Autodesk Inventor part; units mm, degrees
(part 2 of 2)
  arc A141 (-26.798, 74.2336) -> (-27.2062, 73.5932) centre (-26.3001, 73.4659) ccw
  arc A142 (-21.4794, 73.1947) -> (-22.0085, 74.2336) centre (-22.7699, 73.1916) ccw
  circle A143 centre (-25.9605, 73.338) radius 0.5161
  line L108 (-27.2062, 73.5932) -> (-27.2062, 72.1245)
  line L109 (-27.2062, 72.1245) -> (-24.3395, 72.1245)
  line L110 (-24.3395, 71.7056) -> (-28.3839, 71.7056)
  line L111 (-24.3395, 72.1245) -> (-24.3395, 71.7056)
  line L112 (-21.4733, 70.5884) -> (-21.4794, 73.1947)
  arc A144 (-23.3243, 25.8454) -> (-25.4322, 25.8454) centre (-24.3782, 17.6506) ccw
  arc A145 (-25.4322, 25.8454) -> (-26.7856, 25.3656) centre (-25.171, 22.9597) ccw
  arc A146 (-21.9961, 25.3656) -> (-23.3243, 25.8454) centre (-23.7019, 22.7218) ccw
  arc A147 (-21.4671, 24.3267) -> (-21.9961, 25.3656) centre (-22.7575, 24.3237) ccw
  arc A148 (-26.7856, 25.3656) -> (-27.1938, 24.7252) centre (-26.2877, 24.5979) ccw
  circle A149 centre (-25.9607, 24.5305) radius 0.545
  line L113 (-27.1938, 24.7252) -> (-27.1938, 23.2566)
  line L114 (-27.1938, 23.2566) -> (-24.3272, 23.2566)
  line L115 (-24.3272, 23.2566) -> (-24.3272, 22.8376)
  line L116 (-21.461, 21.7204) -> (-21.4671, 24.3267)
  line L117 (-26.0801, 20.1743) -> (-23.0926, 20.1813)
  arc A150 (-22.5618, 19.8544) -> (-21.3196, 20.5365) centre (-22.5875, 21.3734) ccw
  arc A151 (-23.0926, 20.1813) -> (-21.461, 21.7204) centre (-22.9431, 21.6573) ccw
  line L118 (-22.5618, 19.8544) -> (-25.5493, 19.8474)
  line L119 (-21.0597, 22.9429) -> (-21.0597, 21.4689)
  arc A152 (-21.3196, 20.5365) -> (-21.0597, 21.4689) centre (-22.9439, 21.4916) ccw
  line L120 (-19.9288, 22.9429) -> (-21.0597, 22.9429)
  arc A153 (-18.7198, 21.9341) -> (-19.9288, 22.9429) centre (-20.2582, 21.3193) ccw
  arc A154 (-18.5273, 18.7011) -> (-18.7198, 21.9341) centre (-23.4893, 20.0279) ccw
  arc A155 (-20.2704, 17.1911) -> (-18.5273, 18.7011) centre (-20.3549, 19.0497) ccw
  arc A156 (-25.5493, 19.8474) -> (-27.181, 18.3083) centre (-25.6988, 18.3715) ccw
  arc A157 (-26.0801, 20.1743) -> (-27.3224, 19.4922) centre (-26.0545, 18.6554) ccw
  line L121 (-24.3272, 22.8376) -> (-28.3715, 22.8376)
  arc A158 (-27.3224, 19.4922) -> (-27.5822, 18.5598) centre (-25.698, 18.5371) ccw
  line L122 (-27.5822, 17.0858) -> (-27.5822, 18.5598)
  arc A159 (-28.3715, 22.8376) -> (-30.1146, 21.3277) centre (-28.287, 20.979) ccw
  line L123 (-28.7131, 17.0858) -> (-27.5822, 17.0858)
  arc A160 (-30.1146, 21.3277) -> (-29.9221, 18.0946) centre (-25.1526, 20.0009) ccw
  arc A161 (-29.9221, 18.0946) -> (-28.7131, 17.0858) centre (-28.3837, 18.7095) ccw
  arc A162 (-25.3176, 14.1834) -> (-23.2097, 14.1834) centre (-24.2637, 22.3782) ccw
  arc A163 (-26.6458, 14.6631) -> (-25.3176, 14.1834) centre (-24.94, 17.307) ccw
  arc A164 (-23.2097, 14.1834) -> (-21.8563, 14.6631) centre (-23.4709, 17.0691) ccw
  arc A165 (-21.8563, 14.6631) -> (-21.4481, 15.3035) centre (-22.3542, 15.4308) ccw
  arc A166 (-27.1749, 15.702) -> (-26.6458, 14.6631) centre (-25.8844, 15.705) ccw
  circle A167 centre (-22.6938, 15.5587) radius 0.5161
  line L124 (-21.4481, 15.3035) -> (-21.4481, 16.7721)
  line L125 (-21.4481, 16.7721) -> (-24.3148, 16.7721)
  line L126 (-24.3148, 17.1911) -> (-20.2704, 17.1911)
  line L127 (-24.3148, 16.7721) -> (-24.3148, 17.1911)
  line L128 (-27.181, 18.3083) -> (-27.1749, 15.702)
  arc A168 (-46.4728, 48.6946) -> (-44.3649, 48.6946) centre (-45.4189, 56.8894) ccw
  arc A169 (-44.3649, 48.6946) -> (-43.0115, 49.1744) centre (-44.6261, 51.5803) ccw
  arc A170 (-47.801, 49.1744) -> (-46.4728, 48.6946) centre (-46.0952, 51.8182) ccw
  arc A171 (-48.33, 50.2133) -> (-47.801, 49.1744) centre (-47.0396, 50.2163) ccw
  arc A172 (-43.0115, 49.1744) -> (-42.6033, 49.8147) centre (-43.5094, 49.9421) ccw
  circle A173 centre (-43.8364, 50.0095) radius 0.545
  line L129 (-42.6033, 49.8147) -> (-42.6033, 51.2834)
  line L130 (-42.6033, 51.2834) -> (-45.4699, 51.2834)
  line L131 (-45.4699, 51.2834) -> (-45.4699, 51.7023)
  line L132 (-48.3361, 52.8196) -> (-48.33, 50.2133)
  line L133 (-43.717, 54.3657) -> (-46.7045, 54.3587)
  arc A174 (-47.2353, 54.6855) -> (-48.4775, 54.0034) centre (-47.2096, 53.1666) ccw
  arc A175 (-46.7045, 54.3587) -> (-48.3361, 52.8196) centre (-46.854, 52.8827) ccw
  line L134 (-47.2353, 54.6855) -> (-44.2478, 54.6925)
  line L135 (-48.7374, 51.5971) -> (-48.7374, 53.0711)
  arc A176 (-48.4775, 54.0034) -> (-48.7374, 53.0711) centre (-46.8532, 53.0484) ccw
  line L136 (-49.8683, 51.5971) -> (-48.7374, 51.5971)
  arc A177 (-51.0773, 52.6058) -> (-49.8683, 51.5971) centre (-49.5389, 53.2207) ccw
  arc A178 (-51.2698, 55.8389) -> (-51.0773, 52.6058) centre (-46.3078, 54.5121) ccw
  arc A179 (-49.5267, 57.3489) -> (-51.2698, 55.8389) centre (-49.4422, 55.4902) ccw
  arc A180 (-44.2478, 54.6925) -> (-42.6161, 56.2317) centre (-44.0983, 56.1685) ccw
  arc A181 (-43.717, 54.3657) -> (-42.4747, 55.0478) centre (-43.7426, 55.8846) ccw
  line L137 (-45.4699, 51.7023) -> (-41.4256, 51.7023)
  arc A182 (-42.4747, 55.0478) -> (-42.2149, 55.9801) centre (-44.0991, 56.0028) ccw
  line L138 (-42.2149, 57.4541) -> (-42.2149, 55.9801)
  arc A183 (-41.4256, 51.7023) -> (-39.6825, 53.2123) centre (-41.5101, 53.561) ccw
  line L139 (-41.084, 57.4541) -> (-42.2149, 57.4541)
  arc A184 (-39.6825, 53.2123) -> (-39.875, 56.4454) centre (-44.6445, 54.5391) ccw
  arc A185 (-39.875, 56.4454) -> (-41.084, 57.4541) centre (-41.4134, 55.8305) ccw
  arc A186 (-44.4795, 60.3566) -> (-46.5874, 60.3566) centre (-45.5334, 52.1618) ccw
  arc A187 (-43.1513, 59.8769) -> (-44.4795, 60.3566) centre (-44.8571, 57.233) ccw
  arc A188 (-46.5874, 60.3566) -> (-47.9408, 59.8769) centre (-46.3262, 57.4709) ccw
  arc A189 (-47.9408, 59.8769) -> (-48.349, 59.2365) centre (-47.4429, 59.1091) ccw
  arc A190 (-42.6222, 58.8379) -> (-43.1513, 59.8769) centre (-43.9127, 58.8349) ccw
  circle A191 centre (-47.1033, 58.9813) radius 0.5161
  line L140 (-48.349, 59.2365) -> (-48.349, 57.7678)
  line L141 (-48.349, 57.7678) -> (-45.4823, 57.7678)
  line L142 (-45.4823, 57.3489) -> (-49.5267, 57.3489)
  line L143 (-45.4823, 57.7678) -> (-45.4823, 57.3489)
  line L144 (-42.6161, 56.2317) -> (-42.6222, 58.8379)
  arc A192 (-32.7536, 52.0983) -> (-30.6456, 52.0983) centre (-31.6996, 60.2931) ccw
  arc A193 (-30.6456, 52.0983) -> (-29.2922, 52.578) centre (-30.9068, 54.984) ccw
  arc A194 (-34.0817, 52.578) -> (-32.7536, 52.0983) centre (-32.3759, 55.2219) ccw
  arc A195 (-34.6108, 53.6169) -> (-34.0817, 52.578) centre (-33.3203, 53.6199) ccw
  arc A196 (-29.2922, 52.578) -> (-28.884, 53.2184) centre (-29.7901, 53.3457) ccw
  circle A197 centre (-30.1171, 53.4131) radius 0.545
  line L145 (-28.884, 53.2184) -> (-28.884, 54.687)
  line L146 (-28.884, 54.687) -> (-31.7507, 54.687)
  line L147 (-31.7507, 54.687) -> (-31.7507, 55.106)
  line L148 (-34.6169, 56.2232) -> (-34.6108, 53.6169)
  line L149 (-29.9978, 57.7693) -> (-32.9852, 57.7623)
  arc A198 (-33.516, 58.0892) -> (-34.7583, 57.4071) centre (-33.4904, 56.5703) ccw
  arc A199 (-32.9852, 57.7623) -> (-34.6169, 56.2232) centre (-33.1347, 56.2864) ccw
  line L150 (-33.516, 58.0892) -> (-30.5285, 58.0962)
  line L151 (-35.0181, 55.0007) -> (-35.0181, 56.4747)
  arc A200 (-34.7583, 57.4071) -> (-35.0181, 56.4747) centre (-33.1339, 56.452) ccw
  line L152 (-36.1491, 55.0007) -> (-35.0181, 55.0007)
  arc A201 (-37.358, 56.0095) -> (-36.1491, 55.0007) centre (-35.8197, 56.6244) ccw
  arc A202 (-37.5506, 59.2426) -> (-37.358, 56.0095) centre (-32.5885, 57.9158) ccw
  arc A203 (-35.8074, 60.7525) -> (-37.5506, 59.2426) centre (-35.7229, 58.8939) ccw
  arc A204 (-30.5285, 58.0962) -> (-28.8969, 59.6353) centre (-30.379, 59.5722) ccw
  arc A205 (-29.9978, 57.7693) -> (-28.7555, 58.4514) centre (-30.0234, 59.2883) ccw
  line L153 (-31.7507, 55.106) -> (-27.7063, 55.106)
  arc A206 (-28.7555, 58.4514) -> (-28.4957, 59.3838) centre (-30.3798, 59.4065) ccw
  line L154 (-28.4957, 60.8578) -> (-28.4957, 59.3838)
  arc A207 (-27.7063, 55.106) -> (-25.9632, 56.616) centre (-27.7908, 56.9646) ccw
  line L155 (-27.3647, 60.8578) -> (-28.4957, 60.8578)
  arc A208 (-25.9632, 56.616) -> (-26.1557, 59.849) centre (-30.9252, 57.9428) ccw
  arc A209 (-26.1557, 59.849) -> (-27.3647, 60.8578) centre (-27.6941, 59.2342) ccw
  arc A210 (-30.7602, 63.7603) -> (-32.8681, 63.7603) centre (-31.8141, 55.5655) ccw
  arc A211 (-29.4321, 63.2805) -> (-30.7602, 63.7603) centre (-31.1378, 60.6367) ccw
  arc A212 (-32.8681, 63.7603) -> (-34.2215, 63.2805) centre (-32.607, 60.8746) ccw
  arc A213 (-34.2215, 63.2805) -> (-34.6298, 62.6401) centre (-33.7236, 62.5128) ccw
  arc A214 (-28.903, 62.2416) -> (-29.4321, 63.2805) centre (-30.1934, 62.2386) ccw
  circle A215 centre (-33.384, 62.3849) radius 0.5161
  line L156 (-34.6298, 62.6401) -> (-34.6298, 61.1715)
  line L157 (-34.6298, 61.1715) -> (-31.7631, 61.1715)
  line L158 (-31.7631, 60.7525) -> (-35.8074, 60.7525)
  line L159 (-31.7631, 61.1715) -> (-31.7631, 60.7525)
  line L160 (-28.8969, 59.6353) -> (-28.903, 62.2416)
  arc A216 (-30.7461, 36.8007) -> (-32.854, 36.8007) centre (-31.8001, 28.6059) ccw
  arc A217 (-32.854, 36.8007) -> (-34.2075, 36.3209) centre (-32.5929, 33.915) ccw
  arc A218 (-29.418, 36.3209) -> (-30.7461, 36.8007) centre (-31.1237, 33.6771) ccw
  arc A219 (-28.8889, 35.282) -> (-29.418, 36.3209) centre (-30.1793, 35.279) ccw
  arc A220 (-34.2075, 36.3209) -> (-34.6157, 35.6806) centre (-33.7095, 35.5532) ccw
  circle A221 centre (-33.3825, 35.4858) radius 0.545
  line L161 (-34.6157, 35.6806) -> (-34.6157, 34.2119)
  line L162 (-34.6157, 34.2119) -> (-31.749, 34.2119)
  line L163 (-31.749, 34.2119) -> (-31.749, 33.793)
  line L164 (-28.8828, 32.6757) -> (-28.8889, 35.282)
  line L165 (-33.5019, 31.1296) -> (-30.5144, 31.1366)
  arc A222 (-29.9837, 30.8098) -> (-28.7414, 31.4919) centre (-30.0093, 32.3287) ccw
  arc A223 (-30.5144, 31.1366) -> (-28.8828, 32.6757) centre (-30.3649, 32.6126) ccw
  line L166 (-29.9837, 30.8098) -> (-32.9712, 30.8028)
  line L167 (-28.4816, 33.8982) -> (-28.4816, 32.4242)
  arc A224 (-28.7414, 31.4919) -> (-28.4816, 32.4242) centre (-30.3657, 32.4469) ccw
  line L168 (-27.3506, 33.8982) -> (-28.4816, 33.8982)
  arc A225 (-26.1416, 32.8895) -> (-27.3506, 33.8982) centre (-27.68, 32.2746) ccw
  arc A226 (-25.9491, 29.6564) -> (-26.1416, 32.8895) centre (-30.9111, 30.9832) ccw
  arc A227 (-27.6922, 28.1464) -> (-25.9491, 29.6564) centre (-27.7767, 30.0051) ccw
  arc A228 (-32.9712, 30.8028) -> (-34.6028, 29.2636) centre (-33.1206, 29.3268) ccw
  arc A229 (-33.5019, 31.1296) -> (-34.7442, 30.4475) centre (-33.4763, 29.6107) ccw
  line L169 (-31.749, 33.793) -> (-35.7933, 33.793)
  arc A230 (-34.7442, 30.4475) -> (-35.004, 29.5152) centre (-33.1198, 29.4925) ccw
  line L170 (-35.004, 28.0412) -> (-35.004, 29.5152)
  arc A231 (-35.7933, 33.793) -> (-37.5365, 32.283) centre (-35.7089, 31.9343) ccw
  line L171 (-36.135, 28.0412) -> (-35.004, 28.0412)
  arc A232 (-37.5365, 32.283) -> (-37.3439, 29.0499) centre (-32.5745, 30.9562) ccw
  arc A233 (-37.3439, 29.0499) -> (-36.135, 28.0412) centre (-35.8056, 29.6648) ccw
  arc A234 (-32.7395, 25.1387) -> (-30.6316, 25.1387) centre (-31.6855, 33.3335) ccw
  arc A235 (-34.0676, 25.6184) -> (-32.7395, 25.1387) centre (-32.3618, 28.2623) ccw
  arc A236 (-30.6316, 25.1387) -> (-29.2781, 25.6184) centre (-30.8927, 28.0244) ccw
  arc A237 (-29.2781, 25.6184) -> (-28.8699, 26.2588) centre (-29.776, 26.3862) ccw
  arc A238 (-34.5967, 26.6574) -> (-34.0676, 25.6184) centre (-33.3062, 26.6604) ccw
  circle A239 centre (-30.1157, 26.514) radius 0.5161
  line L172 (-28.8699, 26.2588) -> (-28.8699, 27.7275)
  line L173 (-28.8699, 27.7275) -> (-31.7366, 27.7275)
  line L174 (-31.7366, 28.1464) -> (-27.6922, 28.1464)
  line L175 (-31.7366, 27.7275) -> (-31.7366, 28.1464)
  line L176 (-34.6028, 29.2636) -> (-34.5967, 26.6574)
  line L177 (-31.7498, 57.9428) -> (-31.7498, 30.9562) construction
  line L178 (-62.5, 44.45) -> (-1, 44.45) construction
  arc A240 (-46.4728, 28.519) -> (-44.3649, 28.519) centre (-45.4189, 36.7139) ccw
  arc A241 (-44.3649, 28.519) -> (-43.0115, 28.9988) centre (-44.6261, 31.4047) ccw
  arc A242 (-41.4256, 31.5268) -> (-39.6825, 33.0368) centre (-41.5101, 33.3854) ccw
  arc A243 (-42.4747, 34.8722) -> (-42.2149, 35.8046) centre (-44.0991, 35.8273) ccw
  arc A244 (-39.6825, 33.0368) -> (-39.875, 36.2698) centre (-44.6445, 34.3636) ccw
  arc A245 (-39.875, 36.2698) -> (-41.084, 37.2786) centre (-41.4134, 35.655) ccw
  line L179 (-41.084, 37.2786) -> (-42.2149, 37.2786)
  line L180 (-42.2149, 37.2786) -> (-42.2149, 35.8046)
  line L181 (-43.717, 34.1901) -> (-46.7045, 34.1831)
  line L182 (-47.2353, 34.51) -> (-44.2478, 34.517)
  line L183 (-45.4823, 37.5923) -> (-45.4823, 37.1733)
  line L184 (-45.4823, 37.1733) -> (-49.5267, 37.1733)
  line L185 (-42.6161, 36.0561) -> (-42.6222, 38.6624)
  line L186 (-48.349, 37.5923) -> (-45.4823, 37.5923)
  circle A246 centre (-47.1033, 38.8057) radius 0.5161
  line L187 (-48.349, 39.0609) -> (-48.349, 37.5923)
  arc A247 (-47.9408, 39.7013) -> (-48.349, 39.0609) centre (-47.4429, 38.9336) ccw
  arc A248 (-46.5874, 40.1811) -> (-47.9408, 39.7013) centre (-46.3262, 37.2954) ccw
  arc A249 (-44.4795, 40.1811) -> (-46.5874, 40.1811) centre (-45.5334, 31.9862) ccw
  arc A250 (-43.1513, 39.7013) -> (-44.4795, 40.1811) centre (-44.8571, 37.0575) ccw
  arc A251 (-42.6222, 38.6624) -> (-43.1513, 39.7013) centre (-43.9127, 38.6594) ccw
  arc A252 (-43.0115, 28.9988) -> (-42.6033, 29.6392) centre (-43.5094, 29.7665) ccw
  circle A253 centre (-43.8364, 29.8339) radius 0.545
  line L188 (-42.6033, 29.6392) -> (-42.6033, 31.1078)
  line L189 (-42.6033, 31.1078) -> (-45.4699, 31.1078)
  line L190 (-45.4699, 31.5268) -> (-41.4256, 31.5268)
  line L191 (-45.4699, 31.1078) -> (-45.4699, 31.5268)
  arc A254 (-43.717, 34.1901) -> (-42.4747, 34.8722) centre (-43.7426, 35.7091) ccw
  arc A255 (-44.2478, 34.517) -> (-42.6161, 36.0561) centre (-44.0983, 35.993) ccw
  arc A256 (-47.801, 28.9988) -> (-46.4728, 28.519) centre (-46.0952, 31.6427) ccw
  arc A257 (-48.33, 30.0377) -> (-47.801, 28.9988) centre (-47.0396, 30.0407) ccw
  line L192 (-48.3361, 32.644) -> (-48.33, 30.0377)
  arc A258 (-47.2353, 34.51) -> (-48.4775, 33.8279) centre (-47.2096, 32.9911) ccw
  arc A259 (-46.7045, 34.1831) -> (-48.3361, 32.644) centre (-46.854, 32.7072) ccw
  line L193 (-48.7374, 31.4215) -> (-48.7374, 32.8955)
  arc A260 (-48.4775, 33.8279) -> (-48.7374, 32.8955) centre (-46.8532, 32.8728) ccw
  arc A261 (-49.5267, 37.1733) -> (-51.2698, 35.6633) centre (-49.4422, 35.3147) ccw
  line L194 (-49.8683, 31.4215) -> (-48.7374, 31.4215)
  arc A262 (-51.0773, 32.4303) -> (-49.8683, 31.4215) centre (-49.5389, 33.0451) ccw
  arc A263 (-51.2698, 35.6633) -> (-51.0773, 32.4303) centre (-46.3078, 34.3366) ccw
  arc A264 (-19.0326, 28.5164) -> (-16.9247, 28.5164) centre (-17.9786, 36.7112) ccw
  arc A265 (-16.9247, 28.5164) -> (-15.5712, 28.9962) centre (-17.1858, 31.4021) ccw
  arc A266 (-13.9853, 31.5241) -> (-12.2422, 33.0341) centre (-14.0698, 33.3828) ccw
  arc A267 (-15.0345, 34.8696) -> (-14.7747, 35.8019) centre (-16.6588, 35.8246) ccw
  arc A268 (-12.2422, 33.0341) -> (-12.4348, 36.2672) centre (-17.2042, 34.3609) ccw
  arc A269 (-12.4348, 36.2672) -> (-13.6437, 37.2759) centre (-13.9731, 35.6523) ccw
  line L195 (-13.6437, 37.2759) -> (-14.7747, 37.2759)
  line L196 (-14.7747, 37.2759) -> (-14.7747, 35.8019)
  line L197 (-16.2768, 34.1875) -> (-19.2643, 34.1805)
  line L198 (-19.795, 34.5073) -> (-16.8075, 34.5143)
  line L199 (-18.0421, 37.5896) -> (-18.0421, 37.1707)
  line L200 (-18.0421, 37.1707) -> (-22.0865, 37.1707)
  line L201 (-15.1759, 36.0535) -> (-15.182, 38.6597)
  line L202 (-20.9088, 37.5896) -> (-18.0421, 37.5896)
  circle A270 centre (-19.663, 38.8031) radius 0.5161
  line L203 (-20.9088, 39.0583) -> (-20.9088, 37.5896)
  arc A271 (-20.5006, 39.6987) -> (-20.9088, 39.0583) centre (-20.0026, 38.931) ccw
  arc A272 (-19.1471, 40.1784) -> (-20.5006, 39.6987) centre (-18.886, 37.2927) ccw
  arc A273 (-17.0392, 40.1784) -> (-19.1471, 40.1784) centre (-18.0932, 31.9836) ccw
  arc A274 (-15.7111, 39.6987) -> (-17.0392, 40.1784) centre (-17.4168, 37.0548) ccw
  arc A275 (-15.182, 38.6597) -> (-15.7111, 39.6987) centre (-16.4725, 38.6567) ccw
  arc A276 (-15.5712, 28.9962) -> (-15.163, 29.6365) centre (-16.0692, 29.7639) ccw
  circle A277 centre (-16.3962, 29.8313) radius 0.545
  line L204 (-15.163, 29.6365) -> (-15.163, 31.1052)
  line L205 (-15.163, 31.1052) -> (-18.0297, 31.1052)
  line L206 (-18.0297, 31.5241) -> (-13.9853, 31.5241)
  line L207 (-18.0297, 31.1052) -> (-18.0297, 31.5241)
  arc A278 (-16.2768, 34.1875) -> (-15.0345, 34.8696) centre (-16.3024, 35.7064) ccw
  arc A279 (-16.8075, 34.5143) -> (-15.1759, 36.0535) centre (-16.6581, 35.9903) ccw
  arc A280 (-20.3607, 28.9962) -> (-19.0326, 28.5164) centre (-18.655, 31.64) ccw
  arc A281 (-20.8898, 30.0351) -> (-20.3607, 28.9962) centre (-19.5993, 30.0381) ccw
  line L208 (-20.8959, 32.6414) -> (-20.8898, 30.0351)
  arc A282 (-19.795, 34.5073) -> (-21.0373, 33.8252) centre (-19.7694, 32.9884) ccw
  arc A283 (-19.2643, 34.1805) -> (-20.8959, 32.6414) centre (-19.4137, 32.7045) ccw
  line L209 (-21.2971, 31.4189) -> (-21.2971, 32.8929)
  arc A284 (-21.0373, 33.8252) -> (-21.2971, 32.8929) centre (-19.413, 32.8702) ccw
  arc A285 (-22.0865, 37.1707) -> (-23.8296, 35.6607) centre (-22.002, 35.312) ccw
  line L210 (-22.4281, 31.4189) -> (-21.2971, 31.4189)
  arc A286 (-23.6371, 32.4276) -> (-22.4281, 31.4189) centre (-22.0987, 33.0425) ccw
  arc A287 (-23.8296, 35.6607) -> (-23.6371, 32.4276) centre (-18.8676, 34.3339) ccw
  arc A288 (-19.0326, 48.6946) -> (-16.9247, 48.6946) centre (-17.9786, 56.8894) ccw
  arc A289 (-16.9247, 48.6946) -> (-15.5712, 49.1744) centre (-17.1858, 51.5803) ccw
  arc A290 (-13.9853, 51.7023) -> (-12.2422, 53.2123) centre (-14.0698, 53.561) ccw
  arc A291 (-15.0345, 55.0478) -> (-14.7747, 55.9801) centre (-16.6588, 56.0028) ccw
  arc A292 (-12.2422, 53.2123) -> (-12.4348, 56.4454) centre (-17.2042, 54.5391) ccw
  arc A293 (-12.4348, 56.4454) -> (-13.6437, 57.4541) centre (-13.9731, 55.8305) ccw
  line L211 (-13.6437, 57.4541) -> (-14.7747, 57.4541)
  line L212 (-14.7747, 57.4541) -> (-14.7747, 55.9801)
  line L213 (-16.2768, 54.3657) -> (-19.2643, 54.3587)
  line L214 (-19.795, 54.6855) -> (-16.8075, 54.6925)
  line L215 (-18.0421, 57.7678) -> (-18.0421, 57.3489)
  line L216 (-18.0421, 57.3489) -> (-22.0865, 57.3489)
  line L217 (-15.1759, 56.2317) -> (-15.182, 58.8379)
  line L218 (-20.9088, 57.7678) -> (-18.0421, 57.7678)
  circle A294 centre (-19.663, 58.9813) radius 0.5161
  line L219 (-20.9088, 59.2365) -> (-20.9088, 57.7678)
  arc A295 (-20.5006, 59.8769) -> (-20.9088, 59.2365) centre (-20.0026, 59.1091) ccw
  arc A296 (-19.1471, 60.3566) -> (-20.5006, 59.8769) centre (-18.886, 57.4709) ccw
  arc A297 (-17.0392, 60.3566) -> (-19.1471, 60.3566) centre (-18.0932, 52.1618) ccw
  arc A298 (-15.7111, 59.8769) -> (-17.0392, 60.3566) centre (-17.4168, 57.233) ccw
  arc A299 (-15.182, 58.8379) -> (-15.7111, 59.8769) centre (-16.4725, 58.8349) ccw
  arc A300 (-15.5712, 49.1744) -> (-15.163, 49.8147) centre (-16.0692, 49.9421) ccw
  circle A301 centre (-16.3962, 50.0095) radius 0.545
  line L220 (-15.163, 49.8147) -> (-15.163, 51.2834)
  line L221 (-15.163, 51.2834) -> (-18.0297, 51.2834)
  line L222 (-18.0297, 51.7023) -> (-13.9853, 51.7023)
  line L223 (-18.0297, 51.2834) -> (-18.0297, 51.7023)
  arc A302 (-16.2768, 54.3657) -> (-15.0345, 55.0478) centre (-16.3024, 55.8846) ccw
  arc A303 (-16.8075, 54.6925) -> (-15.1759, 56.2317) centre (-16.6581, 56.1685) ccw
  arc A304 (-20.3607, 49.1744) -> (-19.0326, 48.6946) centre (-18.655, 51.8182) ccw
  arc A305 (-20.8898, 50.2133) -> (-20.3607, 49.1744) centre (-19.5993, 50.2163) ccw
  line L224 (-20.8959, 52.8196) -> (-20.8898, 50.2133)
  arc A306 (-19.795, 54.6855) -> (-21.0373, 54.0034) centre (-19.7694, 53.1666) ccw
  arc A307 (-19.2643, 54.3587) -> (-20.8959, 52.8196) centre (-19.4137, 52.8827) ccw
  line L225 (-21.2971, 51.5971) -> (-21.2971, 53.0711)
  arc A308 (-21.0373, 54.0034) -> (-21.2971, 53.0711) centre (-19.413, 53.0484) ccw
  arc A309 (-22.0865, 57.3489) -> (-23.8296, 55.8389) centre (-22.002, 55.4902) ccw
  line L226 (-22.4281, 51.5971) -> (-21.2971, 51.5971)
  arc A310 (-23.6371, 52.6058) -> (-22.4281, 51.5971) centre (-22.0987, 53.2207) ccw
  arc A311 (-23.8296, 55.8389) -> (-23.6371, 52.6058) centre (-18.8676, 54.5121) ccw
  line L227 (-54.8759, 75.4752) -> (-59.8324, 75.4752)
  line L228 (-59.8324, 75.4752) -> (-59.8324, 76.5126)
  line L229 (-59.8324, 76.5126) -> (-57.9881, 76.5126)
  line L230 (-57.9881, 76.5126) -> (-57.9881, 83.3216)
  line L231 (-57.9881, 83.3216) -> (-59.8324, 83.3216)
  line L232 (-59.8324, 83.3216) -> (-59.8324, 84.252)
  spline S0 degree 2 poles (-59.8324, 84.252) (-58.7868, 84.252) (-57.7988, 84.8448) (-57.7329, 85.6682) knots 0 0 0 1 2 2 2
  line L233 (-57.7329, 85.6682) -> (-56.679, 85.6682)
  line L234 (-56.679, 85.6682) -> (-56.679, 76.5126)
  line L235 (-56.679, 76.5126) -> (-54.8759, 76.5126)
  line L236 (-54.8759, 76.5126) -> (-54.8759, 75.4752)
  spline S1 degree 2 poles (-46.6837, 80.5552) (-46.6837, 77.8217) (-48.2727, 75.2612) (-49.9276, 75.2612) knots 0 0 0 1 2 2 2
  spline S2 degree 2 poles (-49.9276, 75.2612) (-51.6073, 75.2612) (-53.1798, 77.8711) (-53.1798, 80.547) knots 0 0 0 1 2 2 2
  spline S3 degree 2 poles (-53.1798, 80.547) (-53.1798, 83.2969) (-51.5908, 85.8411) (-49.9276, 85.8411) knots 0 0 0 1 2 2 2
  spline S4 degree 2 poles (-49.9276, 85.8411) (-48.2563, 85.8411) (-46.6837, 83.2064) (-46.6837, 80.5552) knots 0 0 0 1 2 2 2
  spline S5 degree 2 poles (-48.4292, 77.4595) (-48.2316, 77.9617) (-48.0669, 79.5096) (-48.0669, 80.5552) knots 0 0 0 1 2 2 2
  spline S6 degree 2 poles (-48.0669, 80.5552) (-48.0669, 81.6009) (-48.2316, 83.1405) (-48.4374, 83.6592) knots 0 0 0 1 2 2 2
  spline S7 degree 2 poles (-48.4374, 83.6592) (-48.6432, 84.1779) (-49.3595, 84.7131) (-49.9276, 84.7131) knots 0 0 0 1 2 2 2
  spline S8 degree 2 poles (-49.9276, 84.7131) (-50.4958, 84.7131) (-51.2285, 84.1779) (-51.4426, 83.6427) knots 0 0 0 1 2 2 2
  spline S9 degree 2 poles (-51.4426, 83.6427) (-51.6484, 83.124) (-51.7966, 81.5432) (-51.7966, 80.547) knots 0 0 0 1 2 2 2
  spline S10 degree 2 poles (-51.7966, 80.547) (-51.7966, 79.4767) (-51.6649, 78.044) (-51.4508, 77.4842) knots 0 0 0 1 2 2 2
  spline S11 degree 2 poles (-51.4508, 77.4842) (-51.2532, 76.9572) (-50.5205, 76.3891) (-49.9276, 76.3891) knots 0 0 0 1 2 2 2
  spline S12 degree 2 poles (-49.9276, 76.3891) (-49.3678, 76.3891) (-48.635, 76.9243) (-48.4292, 77.4595) knots 0 0 0 1 2 2 2
  line L237 (-8.6241, 13.7693) -> (-3.6676, 13.7693)
  line L238 (-3.6676, 13.7693) -> (-3.6676, 12.7319)
  line L239 (-3.6676, 12.7319) -> (-5.5119, 12.7319)
  line L240 (-5.5119, 12.7319) -> (-5.5119, 5.9229)
  line L241 (-5.5119, 5.9229) -> (-3.6676, 5.9229)
  line L242 (-3.6676, 5.9229) -> (-3.6676, 4.9926)
  spline S13 degree 2 poles (-3.6676, 4.9926) (-4.7132, 4.9926) (-5.7012, 4.3998) (-5.7671, 3.5764) knots 0 0 0 1 2 2 2
  line L243 (-5.7671, 3.5764) -> (-6.821, 3.5764)
  line L244 (-6.821, 3.5764) -> (-6.821, 12.7319)
  line L245 (-6.821, 12.7319) -> (-8.6241, 12.7319)
  line L246 (-8.6241, 12.7319) -> (-8.6241, 13.7693)
  spline S14 degree 2 poles (-16.8163, 8.6893) (-16.8163, 11.4228) (-15.2273, 13.9834) (-13.5724, 13.9834) knots 0 0 0 1 2 2 2
  spline S15 degree 2 poles (-13.5724, 13.9834) (-11.8927, 13.9834) (-10.3202, 11.3734) (-10.3202, 8.6976) knots 0 0 0 1 2 2 2
  spline S16 degree 2 poles (-10.3202, 8.6976) (-10.3202, 5.9476) (-11.9092, 3.4035) (-13.5724, 3.4035) knots 0 0 0 1 2 2 2
  spline S17 degree 2 poles (-13.5724, 3.4035) (-15.2437, 3.4035) (-16.8163, 6.0382) (-16.8163, 8.6893) knots 0 0 0 1 2 2 2
  spline S18 degree 2 poles (-15.0708, 11.7851) (-15.2684, 11.2829) (-15.4331, 9.735) (-15.4331, 8.6893) knots 0 0 0 1 2 2 2
  spline S19 degree 2 poles (-15.4331, 8.6893) (-15.4331, 7.6437) (-15.2684, 6.1041) (-15.0626, 5.5854) knots 0 0 0 1 2 2 2
  spline S20 degree 2 poles (-15.0626, 5.5854) (-14.8568, 5.0667) (-14.1405, 4.5315) (-13.5724, 4.5315) knots 0 0 0 1 2 2 2
  spline S21 degree 2 poles (-13.5724, 4.5315) (-13.0042, 4.5315) (-12.2715, 5.0667) (-12.0574, 5.6018) knots 0 0 0 1 2 2 2
  spline S22 degree 2 poles (-12.0574, 5.6018) (-11.8516, 6.1205) (-11.7034, 7.7013) (-11.7034, 8.6976) knots 0 0 0 1 2 2 2
  spline S23 degree 2 poles (-11.7034, 8.6976) (-11.7034, 9.7679) (-11.8351, 11.2005) (-12.0492, 11.7604) knots 0 0 0 1 2 2 2
  spline S24 degree 2 poles (-12.0492, 11.7604) (-12.2468, 12.2873) (-12.9795, 12.8554) (-13.5724, 12.8554) knots 0 0 0 1 2 2 2
  spline S25 degree 2 poles (-13.5724, 12.8554) (-14.1322, 12.8554) (-14.865, 12.3203) (-15.0708, 11.7851) knots 0 0 0 1 2 2 2
  line L247 (-54.8759, 75.4752) -> (-59.8324, 75.4752)
  line L248 (-59.8324, 75.4752) -> (-59.8324, 76.5126)
  line L249 (-59.8324, 76.5126) -> (-57.9881, 76.5126)
  line L250 (-57.9881, 76.5126) -> (-57.9881, 83.3216)
  line L251 (-57.9881, 83.3216) -> (-59.8324, 83.3216)
  line L252 (-59.8324, 83.3216) -> (-59.8324, 84.252)
  spline S26 degree 2 poles (-59.8324, 84.252) (-58.7868, 84.252) (-57.7988, 84.8448) (-57.7329, 85.6682) knots 0 0 0 1 2 2 2
  line L253 (-57.7329, 85.6682) -> (-56.679, 85.6682)
  line L254 (-56.679, 85.6682) -> (-56.679, 76.5126)
  line L255 (-56.679, 76.5126) -> (-54.8759, 76.5126)
  line L256 (-54.8759, 76.5126) -> (-54.8759, 75.4752)
  spline S27 degree 2 poles (-46.6837, 80.5552) (-46.6837, 77.8217) (-48.2727, 75.2612) (-49.9276, 75.2612) knots 0 0 0 1 2 2 2
  spline S28 degree 2 poles (-49.9276, 75.2612) (-51.6073, 75.2612) (-53.1798, 77.8711) (-53.1798, 80.547) knots 0 0 0 1 2 2 2
  spline S29 degree 2 poles (-53.1798, 80.547) (-53.1798, 83.2969) (-51.5908, 85.8411) (-49.9276, 85.8411) knots 0 0 0 1 2 2 2
  spline S30 degree 2 poles (-49.9276, 85.8411) (-48.2563, 85.8411) (-46.6837, 83.2064) (-46.6837, 80.5552) knots 0 0 0 1 2 2 2
  spline S31 degree 2 poles (-48.4292, 77.4595) (-48.2316, 77.9617) (-48.0669, 79.5096) (-48.0669, 80.5552) knots 0 0 0 1 2 2 2
  spline S32 degree 2 poles (-48.0669, 80.5552) (-48.0669, 81.6009) (-48.2316, 83.1405) (-48.4374, 83.6592) knots 0 0 0 1 2 2 2
  spline S33 degree 2 poles (-48.4374, 83.6592) (-48.6432, 84.1779) (-49.3595, 84.7131) (-49.9276, 84.7131) knots 0 0 0 1 2 2 2
  spline S34 degree 2 poles (-49.9276, 84.7131) (-50.4958, 84.7131) (-51.2285, 84.1779) (-51.4426, 83.6427) knots 0 0 0 1 2 2 2
  spline S35 degree 2 poles (-51.4426, 83.6427) (-51.6484, 83.124) (-51.7966, 81.5432) (-51.7966, 80.547) knots 0 0 0 1 2 2 2
  spline S36 degree 2 poles (-51.7966, 80.547) (-51.7966, 79.4767) (-51.6649, 78.044) (-51.4508, 77.4842) knots 0 0 0 1 2 2 2
  spline S37 degree 2 poles (-51.4508, 77.4842) (-51.2532, 76.9572) (-50.5205, 76.3891) (-49.9276, 76.3891) knots 0 0 0 1 2 2 2
  spline S38 degree 2 poles (-49.9276, 76.3891) (-49.3678, 76.3891) (-48.635, 76.9243) (-48.4292, 77.4595) knots 0 0 0 1 2 2 2
  line L257 (-8.6241, 13.7693) -> (-3.6676, 13.7693)
  line L258 (-3.6676, 13.7693) -> (-3.6676, 12.7319)
  line L259 (-3.6676, 12.7319) -> (-5.5119, 12.7319)
  line L260 (-5.5119, 12.7319) -> (-5.5119, 5.9229)
  line L261 (-5.5119, 5.9229) -> (-3.6676, 5.9229)
  line L262 (-3.6676, 5.9229) -> (-3.6676, 4.9926)
  spline S39 degree 2 poles (-3.6676, 4.9926) (-4.7132, 4.9926) (-5.7012, 4.3998) (-5.7671, 3.5764) knots 0 0 0 1 2 2 2
  line L263 (-5.7671, 3.5764) -> (-6.821, 3.5764)
  line L264 (-6.821, 3.5764) -> (-6.821, 12.7319)
  line L265 (-6.821, 12.7319) -> (-8.6241, 12.7319)
  line L266 (-8.6241, 12.7319) -> (-8.6241, 13.7693)
  spline S40 degree 2 poles (-16.8163, 8.6893) (-16.8163, 11.4228) (-15.2273, 13.9834) (-13.5724, 13.9834) knots 0 0 0 1 2 2 2
  spline S41 degree 2 poles (-13.5724, 13.9834) (-11.8927, 13.9834) (-10.3202, 11.3734) (-10.3202, 8.6976) knots 0 0 0 1 2 2 2
  spline S42 degree 2 poles (-10.3202, 8.6976) (-10.3202, 5.9476) (-11.9092, 3.4035) (-13.5724, 3.4035) knots 0 0 0 1 2 2 2
  spline S43 degree 2 poles (-13.5724, 3.4035) (-15.2437, 3.4035) (-16.8163, 6.0382) (-16.8163, 8.6893) knots 0 0 0 1 2 2 2
  spline S44 degree 2 poles (-15.0708, 11.7851) (-15.2684, 11.2829) (-15.4331, 9.735) (-15.4331, 8.6893) knots 0 0 0 1 2 2 2
  spline S45 degree 2 poles (-15.4331, 8.6893) (-15.4331, 7.6437) (-15.2684, 6.1041) (-15.0626, 5.5854) knots 0 0 0 1 2 2 2
  spline S46 degree 2 poles (-15.0626, 5.5854) (-14.8568, 5.0667) (-14.1405, 4.5315) (-13.5724, 4.5315) knots 0 0 0 1 2 2 2
  spline S47 degree 2 poles (-13.5724, 4.5315) (-13.0042, 4.5315) (-12.2715, 5.0667) (-12.0574, 5.6018) knots 0 0 0 1 2 2 2
  spline S48 degree 2 poles (-12.0574, 5.6018) (-11.8516, 6.1205) (-11.7034, 7.7013) (-11.7034, 8.6976) knots 0 0 0 1 2 2 2
  spline S49 degree 2 poles (-11.7034, 8.6976) (-11.7034, 9.7679) (-11.8351, 11.2005) (-12.0492, 11.7604) knots 0 0 0 1 2 2 2
  spline S50 degree 2 poles (-12.0492, 11.7604) (-12.2468, 12.2873) (-12.9795, 12.8554) (-13.5724, 12.8554) knots 0 0 0 1 2 2 2
  spline S51 degree 2 poles (-13.5724, 12.8554) (-14.1322, 12.8554) (-14.865, 12.3203) (-15.0708, 11.7851) knots 0 0 0 1 2 2 2
  point P0 (-39.1737, 68.8958)
  point P1 (-39.1737, 20.0009)
  point P2 (-53.7479, 68.8958)
  point P3 (-9.7521, 20.0042)
  point P4 (-13.4723, 102.9238)
  point P5 (-39.1737, 68.8958)
  point P6 (-39.1737, 20.0009)
  point P7 (-53.7479, 68.8958)
  point P8 (-9.7521, 20.0042)
  point P9 (-24.3263, 68.8958)
  point P10 (-24.3272, 68.8958)
  point P11 (-24.3272, 20.0009)
  point P12 (-24.3272, 68.8958)
  point P13 (-24.3272, 20.0009)
  point P14 (-45.4699, 54.5391)
  point P15 (-45.4699, 54.5391)
  point P16 (-45.4699, 54.5391)
  point P17 (-45.4699, 54.5391)
  point P18 (-31.7504, 57.9429)
  point P19 (-31.7507, 57.9428)
  point P20 (-31.7504, 30.9571)
  point P21 (-31.749, 30.9562)
  point P22 (-18.0297, 54.5391)
  point P23 (-45.4699, 34.3609)
  point P24 (-18.0297, 34.3609)
  point P25 (-45.4699, 34.3636)
  point P26 (-45.4699, 34.3636)
  point P27 (-45.4699, 34.3636)
  point P28 (-45.4699, 34.3636)
  point P29 (-18.0297, 34.3609)
  point P30 (-18.0297, 34.3609)
  point P31 (-18.0297, 34.3609)
  point P32 (-18.0297, 34.3609)
  point P33 (-18.0297, 54.5391)
  point P34 (-18.0297, 54.5391)
  point P35 (-18.0297, 54.5391)
  point P36 (-18.0297, 54.5391)
  dimension "d103" = 8.4153
  dimension "d105" = 0.508
  dimension "d106" = 0.508
  constraints: 572 point on circle, 428 end point, 312 centre point, 52 perpendicular, 52 tangent, 21 vertical, 10 horizontal, 3 symmetric about line, 2 midpoint, 1 parallel, 5 other
  measures "d103" distance of L11.end L13.start
  measures "d105" distance between parallel lines of L14 L6
  measures "d106" distance between parallel lines of L15 L10
extrude "Extrusion20" add sketch "Sketch17" along normal blind 0.4 contours A112 L94 L95 A116 A117 A115 L92 L2 | L2 L92 L88 L90 L93 A111 A110 A108 A114 A109 L89 A107 L91 A113 A112 | L245 L246 L237 L2 | L2 L237 L238 L239 L240 L241 L242 S13 L243 L244 L245 | L39 A34 A33 A32 L38 L37 L36 L35 A31 A30 A29 A28 A27 L34 A26 L33 A25 A24 L32 | L55 A58 A57 A56 L54 L53 L52 L51 A55 A54 A53 A52 A51 L50 A50 L49 A49 A48 L48 | L71 A82 A81 A80 L70 L69 L68 L67 A79 A78 A77 A76 A75 L66 A74 L65 A73 A72 L64 | A122 A123 L100 A127 L101 A133 A134 L106 L107 A137 A136 A135 L105 L99 L98 L97 A124 A121 A120 | A150 A152 L119 L120 A153 A154 A155 L126 L127 L125 L124 A165 A164 A162 A163 A166 L128 A156 L118 | A174 A176 L135 L136 A177 A178 A179 L142 L143 L141 L140 A189 A188 A186 A187 A190 L144 A180 L134 | A198 A200 L151 L152 A201 A202 A203 L158 L159 L157 L156 A213 A212 A210 A211 A214 L160 A204 L150 | A222 A224 L167 L168 A225 A226 A227 L174 L175 L173 L172 A237 A236 A234 A235 A238 L176 A228 L166 | A256 A257 L192 A259 L181 A254 A243 L180 L179 A245 A244 A242 L190 L191 L189 L188 A252 A241 A240 | A280 A281 L208 A283 L197 A278 A267 L196 L195 A269 A268 A266 L206 L207 L205 L204 A276 A265 A264 | A306 A308 L225 L226 A310 A311 A309 L216 L215 L218 L219 A295 A296 A297 A298 A299 L217 A303 L214 | L227 L228 L229 L230 L231 L232 S0 L233 L234 L235 L236 | S1 S2 S3 S4 | S14 S15 S16 S17 bodies 1
sketch "Sketch18" plane through (0, 0, -0.2) normal (0, 0, -1) x (-1, 0, 0)
  line L0 (0, 0) -> (-63.5, 0)
  line L1 (-63.5, 0) -> (-63.5, 88.9)
  line L2 (-63.5, 88.9) -> (0, 88.9)
  line L3 (0, 88.9) -> (0, 0)
  constraints: 8 end point, 2 parallel, 1 horizontal, 1 perpendicular
extrude "Extrusion21" add sketch "Sketch18" along normal blind 0.4 bodies 3
fillet "Fillet2" radius 3.175 8 edges at (63.5, 0, 0.2) (63.5, 88.9, 0.2) (0, 0, 0.2) (0, 88.9, 0.2) (63.5, 0, -0.3) (63.5, 88.9, -0.3) (0, 0, -0.3) (0, 88.9, -0.3)
extrude "Extrusion22" cut sketch "Sketch17" along normal blind 0.4 contours A112 L94 L95 A116 A117 A115 L92 L2 | L2 L92 L88 L90 L93 A111 A110 A108 A114 A109 L89 A107 L91 A113 A112 | L245 L246 L237 L2 | L2 L237 L238 L239 L240 L241 L242 S13 L243 L244 L245 | L39 A34 A33 A32 L38 L37 L36 L35 A31 A30 A29 A28 A27 L34 A26 L33 A25 A24 L32 | L43 A41 A40 L46 L47 A44 A45 A43 L44 L40 L42 L45 A39 A38 A36 A42 A37 L41 A35 | L55 A58 A57 A56 L54 L53 L52 L51 A55 A54 A53 A52 A51 L50 A50 L49 A49 A48 L48 | L59 A65 A64 L62 L63 A68 A69 A67 L60 L56 L58 L61 A63 A62 A60 A66 A61 L57 A59 | L71 A82 A81 A80 L70 L69 L68 L67 A79 A78 A77 A76 A75 L66 A74 L65 A73 A72 L64 | L75 A89 A88 L78 L79 A92 A93 A91 L76 L72 L74 L77 A87 A86 A84 A90 A85 L73 A83 | L87 A106 A105 A104 L86 L85 L84 L83 A103 A102 A101 A100 A99 L82 A98 L81 A97 A96 L80 | A122 A123 L100 A127 L101 A133 A134 L106 L107 A137 A136 A135 L105 L99 L98 L97 A124 A121 A120 | A126 A128 L103 L104 A129 A130 A131 L110 L111 L109 L108 A141 A140 A138 A139 A142 L112 A132 L102 | A146 A147 L116 A151 L117 A157 A158 L122 L123 A161 A160 A159 L121 L115 L114 L113 A148 A145 A144 | A150 A152 L119 L120 A153 A154 A155 L126 L127 L125 L124 A165 A164 A162 A163 A166 L128 A156 L118 | A170 A171 L132 A175 L133 A181 A182 L138 L139 A185 A184 A183 L137 L131 L130 L129 A172 A169 A168 | A174 A176 L135 L136 A177 A178 A179 L142 L143 L141 L140 A189 A188 A186 A187 A190 L144 A180 L134 | A194 A195 L148 A199 L149 A205 A206 L154 L155 A209 A208 A207 L153 L147 L146 L145 A196 A193 A192 | A198 A200 L151 L152 A201 A202 A203 L158 L159 L157 L156 A213 A212 A210 A211 A214 L160 A204 L150 | A218 A219 L164 A223 L165 A229 A230 L170 L171 A233 A232 A231 L169 L163 L162 L161 A220 A217 A216 | A222 A224 L167 L168 A225 A226 A227 L174 L175 L173 L172 A237 A236 A234 A235 A238 L176 A228 L166 | A256 A257 L192 A259 L181 A254 A243 L180 L179 A245 A244 A242 L190 L191 L189 L188 A252 A241 A240 | A258 A260 L193 L194 A262 A263 A261 L184 L183 L186 L187 A247 A248 A249 A250 A251 L185 A255 L182 | A280 A281 L208 A283 L197 A278 A267 L196 L195 A269 A268 A266 L206 L207 L205 L204 A276 A265 A264 | A282 A284 L209 L210 A286 A287 A285 L200 L199 L202 L203 A271 A272 A273 A274 A275 L201 A279 L198 | A304 A305 L224 A307 L213 A302 A291 L212 L211 A293 A292 A290 L222 L223 L221 L220 A300 A289 A288 | A306 A308 L225 L226 A310 A311 A309 L216 L215 L218 L219 A295 A296 A297 A298 A299 L217 A303 L214 | L227 L228 L229 L230 L231 L232 S0 L233 L234 L235 L236 | S1 S2 S3 S4 | S14 S15 S16 S17 bodies 3
extrude "Extrusion23" add sketch "Sketch17" along normal blind 0.4 contours L43 A41 A40 L46 L47 A44 A45 A43 L44 L40 L42 L45 A39 A38 A36 A42 A37 L41 A35 | L59 A65 A64 L62 L63 A68 A69 A67 L60 L56 L58 L61 A63 A62 A60 A66 A61 L57 A59 | L75 A89 A88 L78 L79 A92 A93 A91 L76 L72 L74 L77 A87 A86 A84 A90 A85 L73 A83 | L87 A106 A105 A104 L86 L85 L84 L83 A103 A102 A101 A100 A99 L82 A98 L81 A97 A96 L80 | A126 A128 L103 L104 A129 A130 A131 L110 L111 L109 L108 A141 A140 A138 A139 A142 L112 A132 L102 | A146 A147 L116 A151 L117 A157 A158 L122 L123 A161 A160 A159 L121 L115 L114 L113 A148 A145 A144 | A170 A171 L132 A175 L133 A181 A182 L138 L139 A185 A184 A183 L137 L131 L130 L129 A172 A169 A168 | A194 A195 L148 A199 L149 A205 A206 L154 L155 A209 A208 A207 L153 L147 L146 L145 A196 A193 A192 | A218 A219 L164 A223 L165 A229 A230 L170 L171 A233 A232 A231 L169 L163 L162 L161 A220 A217 A216 | A258 A260 L193 L194 A262 A263 A261 L184 L183 L186 L187 A247 A248 A249 A250 A251 L185 A255 L182 | A282 A284 L209 L210 A286 A287 A285 L200 L199 L202 L203 A271 A272 A273 A274 A275 L201 A279 L198 | A304 A305 L224 A307 L213 A302 A291 L212 L211 A293 A292 A290 L222 L223 L221 L220 A300 A289 A288 bodies 4
